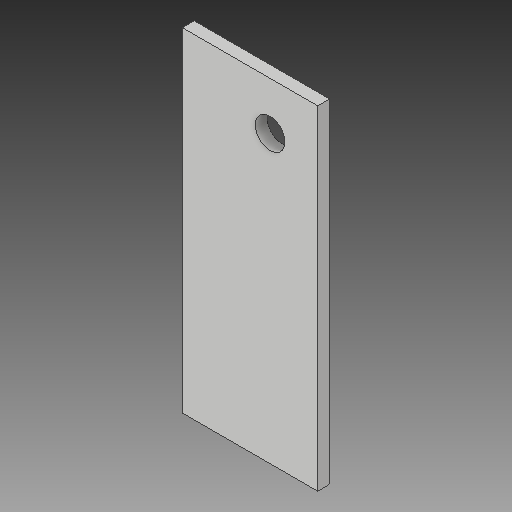
# Autodesk Inventor part: polycarb wall for saw blade
Saved by Autodesk Inventor 2019 (Build 230136000, 136)
## iProperties
Created: 2018-01-09
Part Number: polycarb wall for saw blade
Material: Generic
Document SubType Name: Modeling
Designer: Administrator
Density: 1 g/cm^3
Appearance: Default
Author: Administrator
Autodesk Inventor part; units mm, degrees
ref_plane "YZ Plane" through (0, 0, 0) normal (1, 0, 0) x (0, 1, 0)
ref_plane "XZ Plane" through (0, 0, 0) normal (0, 1, 0) x (-1, 0, 0)
ref_plane "XY Plane" through (0, 0, 0) normal (0, 0, 1) x (1, 0, 0)
sketch "Sketch1" plane through (0, 0, 0) normal (0, 0, 1) x (1, 0, 0)
  line L0 (0, 0) -> (50.8, 0)
  line L1 (50.8, 0) -> (50.8, 190.5)
  line L2 (50.8, 190.5) -> (0, 190.5)
  line L3 (0, 190.5) -> (0, 0)
  dimension "d0" = 50.8
  dimension "d1" = 190.5
  constraints: 8 end point, 2 parallel, 1 horizontal, 1 perpendicular
  measures "d0" distance of L0.start L0.end
  measures "d1" distance of L0.end L1.end
extrude "Extrusion1" add sketch "Sketch1" along normal blind 6.35
sketch "Sketch2" plane through (0, 0, 6.35) normal (0, 0, 1) x (1, 0, 0)
  circle A0 centre (36.0934, 152.4) radius 7.9375
  line L0 (0, 0) -> (50.8, 0) projected
  line L1 (50.8, 0) -> (50.8, 190.5) projected
  dimension "d4" = 152.4
  dimension "d5" = 15.875
  dimension "d15" = 14.7066
  constraints: 1 centre point
  measures "d4" distance from line of L0 A0.centre
  measures "d5" diameter of A0
  measures "d15" distance from line of L1 A0.centre
extrude "Extrusion2" cut sketch "Sketch2" against normal blind 6.35
sketch "Sketch3" plane through (0, 0, 6.35) normal (0, 0, 1) x (1, 0, 0)
  line L0 (0, 190.5) -> (0, 0) projected
  line L1 (50.8, 0) -> (50.8, 190.5) projected
  line L2 (0, 177.8) -> (50.8, 177.8)
  line L3 (50.8, 177.8) -> (50.8, 190.5)
  line L4 (50.8, 190.5) -> (0, 190.5)
  line L5 (0, 190.5) -> (0, 177.8)
  dimension "d8" = 12.7
  constraints: 8 end point, 2 parallel, 1 horizontal, 1 perpendicular, 1 point on line
  measures "d8" distance between parallel lines of L4 L2
extrude "Extrusion3" cut sketch "Sketch3" against normal blind 25.4
sketch "Sketch4" plane through (0, 0, 6.35) normal (0, 0, 1) x (1, 0, 0)
  line L0 (0, 0) -> (50.8, 0) projected
  line L1 (0, 0) -> (-10.6807, 0)
  line L2 (-10.6807, 0) -> (-10.6807, 177.8)
  line L3 (-10.6807, 177.8) -> (0, 177.8)
  line L4 (0, 177.8) -> (0, 0)
  line L5 (50.8, 0) -> (61.4807, 0)
  line L6 (61.4807, 0) -> (61.4807, 177.8)
  line L7 (61.4807, 177.8) -> (50.8, 177.8)
  line L8 (50.8, 177.8) -> (50.8, 0)
  dimension "d11" = 10.6807
  dimension "d12" = 10.6807
  constraints: 16 end point, 4 parallel, 2 horizontal, 2 perpendicular
  measures "d11" distance of L2.end L3.end
  measures "d12" distance of L6.end L7.end
extrude "Extrusion4" add sketch "Sketch4" against normal blind 6.35
body "Solid1"
